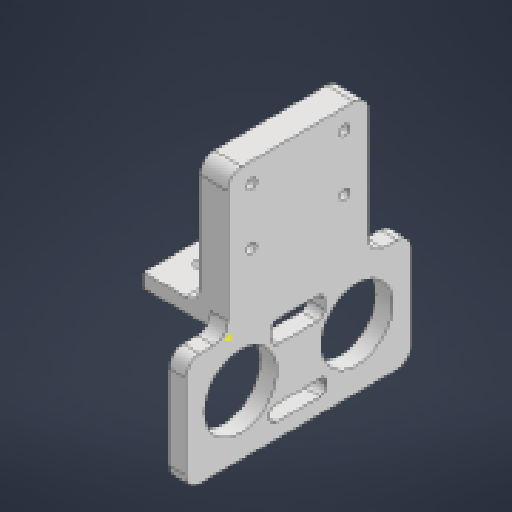
# Autodesk Inventor part: Camera Mount
Saved by Autodesk Inventor 2023 (Build 270158000, 158)
## iProperties
Created: 2023-01-22
Part Number: Camera Mount
Material: Generic
Document SubType Name: Modeling
Designer: Michael
Density: 1 g/cm^3
Appearance: Default
Author: Michael
Autodesk Inventor part; units mm, degrees
ref_plane "YZ Plane" through (0, 0, 0) normal (1, 0, 0) x (0, 1, 0)
ref_plane "XZ Plane" through (0, 0, 0) normal (0, 1, 0) x (-1, 0, 0)
ref_plane "XY Plane" through (0, 0, 0) normal (0, 0, 1) x (1, 0, 0)
sketch "Sketch1" plane through (0, 0, 0) normal (1, 0, 0) x (0, 1, 0)
  line L0 (0, 0) -> (31.75, 0)
  line L1 (31.75, 0) -> (31.75, -31.75)
  line L2 (31.75, -31.75) -> (0, -31.75)
  line L3 (0, -31.75) -> (0, 0)
  dimension "d0" = 31.75
  dimension "d1" = 31.75
  constraints: 8 end point, 2 parallel, 1 horizontal, 1 perpendicular
  measures "d0" distance of L1.end L2.end
  measures "d1" distance of L0.end L1.end
extrude "Extrusion1" add sketch "Sketch1" along normal blind 6.35
sketch "Sketch3" plane through (0, 0, -31.75) normal (0, -1, 0) x (1, 0, 0)
  line L0 (0, 31.75) -> (6.35, 31.75) projected
  line L1 (0, 31.75) -> (-12.7, 31.75)
  line L2 (-12.7, 31.75) -> (-12.7, 0)
  line L3 (-12.7, 0) -> (0, 0)
  line L4 (0, 0) -> (0, 31.75)
  dimension "d10" = 12.7
  constraints: 8 end point, 2 parallel, 1 horizontal, 1 perpendicular
  measures "d10" distance of L3.end L2.end
extrude "Extrusion3" add sketch "Sketch3" against normal blind 3.175
fillet "Fillet1" radius 3.175 1 edges at (0, 3.175, -15.875)
fillet "Fillet2" radius 3.175 2 edges at (3.175, 31.75, -31.75) (3.175, 31.75, 0)
sketch "Sketch4" plane through (0, 3.175, -31.75) normal (0, 1, 0) x (1, 0, 0)
  line L0 (-3.175, 0) -> (-3.175, -31.75) projected
  line L1 (-3.175, 0) -> (-12.7, 0) projected
  line L2 (-12.7, 0) -> (-12.7, -31.75) projected
  line L3 (-12.7, -31.75) -> (-3.175, -31.75) projected
  line L4 (-12.7, -15.875) -> (-3.175, -15.875)
  line L5 (-12.7, -31.75) -> (6.35, -31.75) projected
  line L6 (-7.9375, -31.75) -> (-7.9375, 0)
  point P0 (0, -31.75)
  point P1 (-7.9375, -23.8125)
  point P2 (-7.9375, -7.9375)
  dimension "d15" = 4.7625
  dimension "d17" = 7.9375
  constraints: 4 end point, 3 midpoint, 1 point on line, 1 symmetric about line
  measures "d15" distance from line of L2 point (-7.938, -23.812)
  measures "d17" distance from line of point (-7.938, -23.812) L3
hole "Hole1" at (-7.9375, 3.175, -7.9375) at (-7.9375, 3.175, -23.8125) direction (0, -1, 0) diameter 2.4 end through all
sketch "Sketch5" plane through (6.35, 0, -31.75) normal (0, -1, 0) x (1, 0, 0)
  line L0 (0, 31.75) -> (0, 0) projected
  line L1 (0, -9.525) -> (-3.81, -9.525)
  line L2 (-3.81, -9.525) -> (-3.81, 41.275)
  line L3 (-3.81, 41.275) -> (0, 41.275)
  line L4 (0, 41.275) -> (0, -9.525)
  line L5 (-19.05, 0) -> (0, 0) projected
  point P0 (-6.35, 31.75)
  point P1 (-1.905, -9.525)
  dimension "d25" = 50.8
  dimension "d26" = 9.525
  dimension "d40" = 3.81
  constraints: 8 end point, 2 parallel, 1 horizontal, 1 midpoint, 1 perpendicular, 1 vertical
  measures "d25" distance of L1.end L2.end
  measures "d26" distance from line of point (-1.905, -9.525) L5
  measures "d40" distance of L2.end L3.end
extrude "Extrusion4" add sketch "Sketch5" along normal blind 25.4
sketch "Sketch6" plane through (6.35, 0, 0) normal (1, 0, 0) x (0, 0, -1)
  circle A0 centre (5.3718, 27.21) radius 1 projected
  circle A1 centre (5.3718, 14.71) radius 1 projected
  circle A2 centre (26.3718, 14.71) radius 1 projected
  circle A3 centre (26.3718, 27.21) radius 1 projected
  point P0 (0, 0)
  constraints: 4 coincident
hole "Hole2" at (6.35, 27.21, -5.3718) at (6.35, 27.21, -26.3718) at (6.35, 14.71, -26.3718) at (6.35, 14.71, -5.3718) direction (-1, 0, 0) diameter 2.2 end through all
sketch "Sketch7" plane through (6.35, 0, 0) normal (1, 0, 0) x (0, 0, -1)
  circle A0 centre (2.8719, -12) radius 8 projected
  arc A1 (11.3719, -2) -> (9.8719, -3.5) centre (11.3719, -3.5) ccw projected
  line L0 (20.3719, -2) -> (11.3719, -2) projected
  arc A2 (21.8719, -3.5) -> (20.3719, -2) centre (20.3719, -3.5) ccw projected
  line L1 (21.8719, -5.5) -> (21.8719, -3.5) projected
  arc A3 (20.3719, -7) -> (21.8719, -5.5) centre (20.3719, -5.5) ccw projected
  line L2 (11.3719, -7) -> (20.3719, -7) projected
  arc A4 (9.8719, -5.5) -> (11.3719, -7) centre (11.3719, -5.5) ccw projected
  line L3 (9.8719, -3.5) -> (9.8719, -5.5) projected
  circle A5 centre (28.8719, -12) radius 8 projected
  line L4 (20.8719, -18.5) -> (10.8719, -18.5) projected
  arc A6 (10.8719, -18.5) -> (9.3719, -20) centre (10.8719, -20) ccw projected
  arc A7 (9.3719, -20.5) -> (10.8719, -22) centre (10.8719, -20.5) ccw projected
  line L5 (9.3719, -20) -> (9.3719, -20.5) projected
  line L6 (10.8719, -22) -> (20.8719, -22) projected
  arc A8 (20.8719, -22) -> (22.3719, -20.5) centre (20.8719, -20.5) ccw projected
  line L7 (22.3719, -20.5) -> (22.3719, -20) projected
  arc A9 (22.3719, -20) -> (20.8719, -18.5) centre (20.8719, -20) ccw projected
  point P0 (0, 0)
extrude "Extrusion6" cut sketch "Sketch7" against normal blind 12.7
fillet "Fillet3" radius 3.175 6 edges at (4.445, 0, 0) (4.445, 0, -31.75) (4.445, 0, -41.275) (4.445, -25.4, -41.275) (4.445, -25.4, 9.525) (4.445, 0, 9.525)
sketch "Sketch12" plane through (6.35, 0, 0) normal (1, 0, 0) x (0, 0, -1)
  circle A0 centre (28.9671, -12.1524) radius 8.5785
  point P0 (0, 0)
  constraints: 1 centre point
extrude "Extrusion11" add sketch "Sketch12" against normal blind 3.81
sketch "Sketch14" plane through (6.35, 0, 0) normal (1, 0, 0) x (0, 0, -1)
  circle A0 centre (29.1119, -12) radius 8
  circle A1 centre (29.1119, -12) radius 8.1524
  circle A2 centre (2.8719, -12) radius 8
  circle A3 centre (2.8719, -12) radius 8.1524
  point P0 (0, 0)
  dimension "d60" = 0.1524
  dimension "d61" = 0.1524
  constraints: 4 centre point, 4 other
  measures "d60" radial gap between concentric circles of A0 A1
  measures "d61" radial gap between concentric circles of A2 A3
extrude "Extrusion13" cut sketch "Sketch14" against normal blind 25.4 contours A0 | A2 | A3
sketch "Sketch15" plane through (6.35, 0, 0) normal (1, 0, 0) x (0, 0, -1)
  point P0 (0, 0)
sketch "Sketch16" plane through (6.35, 0, 0) normal (1, 0, 0) x (0, 0, -1)
  line L0 (19.9133, 16.7444) -> (19.9133, 22.2444)
  line L1 (18.4133, 23.7444) -> (12.9133, 23.7444)
  line L2 (11.4133, 22.2444) -> (11.4133, 16.7444)
  line L3 (12.9133, 15.2444) -> (18.4133, 15.2444)
  line L4 (19.9133, 23.7444) -> (11.4133, 23.7444)
  line L5 (11.4133, 23.7444) -> (11.4133, 15.2444)
  line L6 (11.4133, 15.2444) -> (19.9133, 15.2444)
  line L7 (19.9133, 15.2444) -> (19.9133, 23.7444)
  line L8 (11.2863, 23.8714) -> (20.0403, 23.8714)
  line L9 (20.0403, 23.8714) -> (20.0403, 15.1174)
  line L10 (20.0403, 15.1174) -> (11.2863, 15.1174)
  line L11 (11.2863, 15.1174) -> (11.2863, 23.8714)
  point P0 (0, 0)
  dimension "d64" = 0.127
  dimension "d65" = 8.754
  constraints: 24 end point, 4 parallel, 3 horizontal, 2 perpendicular, 2 vertical, 11 other
  measures "d64" distance between parallel lines of L4 L8
  measures "d65" distance of L8.start L8.end
extrude "Extrusion14" cut sketch "Sketch16" against normal blind 25.4 contours L7 L6 L3 L5 L2 L4 L1 L0 | L8 L9 L10 L11
body "Solid1"
